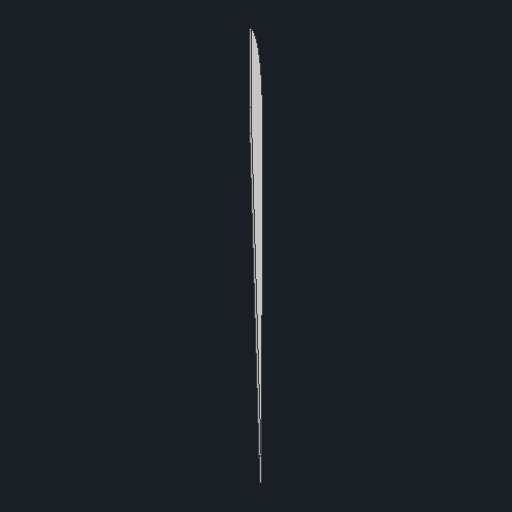
# Autodesk Inventor part: standoff
Saved by Autodesk Inventor 2023 (Build 270158030, 158C)
## iProperties
Created: 2022-03-24
Part Number: standoff
Material: Generic
Document SubType Name: Modeling
Designer: kardo
Density: 1 g/cm^3
Appearance: Default
Author: kardo
Autodesk Inventor part; units mm, degrees
ref_plane "YZ Plane" through (0, 0, 0) normal (1, 0, 0) x (0, 1, 0)
ref_plane "XZ Plane" through (0, 0, 0) normal (0, 1, 0) x (-1, 0, 0)
ref_plane "XY Plane" through (0, 0, 0) normal (0, 0, 1) x (1, 0, 0)
derived "parameters_frame.ipt"
derived "surface_body.ipt"
sketch "sk_rail_bottom_standoff" plane through (34.32, 0, 0) normal (1, 0, 0) x (0, 1, 0)
  line L0 (-363, 18.496) -> (-275.8801, 19.4795)
  arc A0 (-275.8801, 19.4795) -> (-254.1001, 19.9549) centre (-287.5515, 1053.3708) ccw
  line L1 (30.81, 28.832) -> (94.8, 28.832)
  arc A1 (30.81, 28.832) -> (9.48, 28.4869) centre (30.81, -630.4631) ccw
  line L2 (-254.1001, 19.9549) -> (9.48, 28.4869)
  line L3 (-483, 0) -> (357, 0) construction
  line L4 (9.48, 28.4869) -> (9.48, 0) construction
  line L5 (-254.1001, 19.9549) -> (-254.1001, 0) construction
  point P0 (0, 0)
  point P1 (-254.1001, 19.7253)
  point P2 (9.48, 28.832)
sketch "sk_rail_standoff_standoff" plane through (34.32, 0, 0) normal (1, 0, 0) x (0, 1, 0)
  line L0 (0, 18.496) -> (77.736, 18.1714) construction
  line L1 (77.736, 18.1714) -> (94.8, 28.832) construction
  line L2 (0, 18.496) -> (-254.1001, 19.5569)
  line L3 (-275.8801, 19.4795) -> (-363, 18.496)
  arc A0 (-254.1001, 19.5569) -> (-275.8801, 19.4795) centre (-259.9809, -1388.9263) ccw
  line L4 (-483, 0) -> (357, 0) construction
  line L5 (-254.1001, 19.5569) -> (-254.1001, 0) construction
  spline S0 degree 2 poles (0, 18.496) (77.736, 18.1714) (94.8, 28.832) knots 1 1 1 2 2 2
  point P0 (0, 0)
  point P1 (-254.1001, 19.7253)
ref_plane "plane_standoff_right" through (34.32, 0, 0) normal (1, 0, 0) x (0, 1, 0)
sketch "sk_base" plane through (34.32, 0, 0) normal (1, 0, 0) x (0, 1, 0)
  arc A0 (-254.1001, 19.5569) -> (-275.8801, 19.4795) centre (-259.9809, -1388.9263) ccw construction
  arc A1 (-275.8801, 19.4795) -> (-254.1001, 19.9549) centre (-287.5515, 1053.3708) ccw construction
  line L0 (-254.1001, 19.9549) -> (9.48, 28.4869) construction
  line L1 (0, 18.496) -> (-254.1001, 19.5569) construction
  spline S0 degree 2 poles (0, 18.496) (77.736, 18.1714) (94.8, 28.832) knots 1 1 1 2 2 2 construction
  line L2 (30.81, 28.832) -> (94.8, 28.832) construction
  arc A2 (30.81, 28.832) -> (9.48, 28.4869) centre (30.81, -630.4631) ccw construction
  line L3 (0.005, 19.696) -> (-254.0951, 20.7569)
  arc A3 (-254.0951, 20.7569) -> (-275.8801, 20.6796) centre (-259.9809, -1388.9263) ccw
  arc A4 (-275.8801, 20.6796) -> (-254.1389, 21.1542) centre (-287.5515, 1053.3708) ccw
  line L4 (-254.1389, 21.1542) -> (9.4412, 29.6862)
  arc A5 (30.81, 30.032) -> (9.4412, 29.6862) centre (30.81, -630.4631) ccw
  line L5 (30.81, 30.032) -> (92.8, 30.032)
  line L6 (-275.8801, 19.4795) -> (-275.8801, 20.6796) construction
  line L7 (92.8, 29.0697) -> (92.8, 30.032)
  spline S1 degree 5 poles (92.8, 29.0697) (91.3593, 28.3123) (89.8548, 27.6759) (88.3268, 27.1138) (84.0606, 25.735) (79.6917, 24.7183) (76.8931, 24.1603) (70.3385, 23.0293) (63.7366, 22.2113) (59.9593, 21.8156) (51.4371, 21.0566) (42.8962, 20.5448) (38.1435, 20.3183) (27.6665, 19.9272) (17.1836, 19.7389) (11.4575, 19.6846) (5.7312, 19.6721) (0.005, 19.696) knots 0 0 0 0 0 0 0.086761 0.086761 0.086761 0.238802 0.238802 0.238802 0.441207 0.441207 0.441207 0.694793 0.694793 0.694793 1 1 1 1 1 1
  point P0 (0, 0)
  dimension "d5" = 1.2
  dimension "d4" = 1.2
  dimension "d6" = 2
  constraints: 10 end point, 6 point on circle, 3 centre point, 2 vertical, 1 parallel, 7 other
  measures "d4" distance between parallel lines of L0 L4
  measures "d6" distance from line of L7 point (94.8, 28.832)
extrude "thicken" add sketch "sk_base" against normal blind 2
equation "\"d4\" = shell_thickness"
equation "\"d6\" = bulkhead_thickness"
equation "\"d2\" = bulkhead_thickness"
equation "\"shell_thickness\" = 1.2"
equation "\"bulkhead_thickness\" = 2"
body "Solid1"
